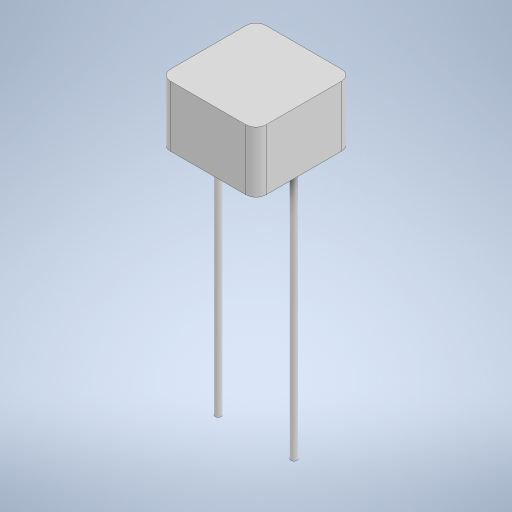
# Autodesk Inventor part: KM6A – H90
Saved by Autodesk Inventor 2024 (Build 280153000, 153)
## iProperties
Created: 2023-12-04
Part Number: KM6A – H90
Material: Типовые
Document SubType Name: Modeling
Designer: SaNe4Ka
Density: 1 g/cm^3
Appearance: По умолчанию
Author: SaNe4Ka
Autodesk Inventor part; units mm, degrees
ref_plane "YZ Plane" through (0, 0, 0) normal (1, 0, 0) x (0, 1, 0)
ref_plane "XZ Plane" through (0, 0, 0) normal (0, 1, 0) x (-1, 0, 0)
ref_plane "XY Plane" through (0, 0, 0) normal (0, 0, 1) x (1, 0, 0)
sketch "Эскиз1" plane through (0, 0, 0) normal (0, 1, 0) x (-1, 0, 0)
  line L0 (5.945, 7.1046) -> (-1.555, 7.1046)
  line L1 (-2.555, 6.1046) -> (-2.555, -1.3954)
  line L2 (-1.555, -2.3954) -> (5.945, -2.3954)
  line L3 (6.945, -1.3954) -> (6.945, 6.1046)
  arc A0 (6.945, 6.1046) -> (5.945, 7.1046) centre (5.945, 6.1046) ccw
  arc A1 (5.945, -2.3954) -> (6.945, -1.3954) centre (5.945, -1.3954) ccw
  arc A2 (-2.555, -1.3954) -> (-1.555, -2.3954) centre (-1.555, -1.3954) ccw
  arc A3 (-1.555, 7.1046) -> (-2.555, 6.1046) centre (-1.555, 6.1046) ccw
  point P0 (0, 0)
  point P1 (-2.555, -2.3954)
  point P2 (-2.555, 7.1046)
  point P3 (6.945, -2.3954)
  dimension "d0" = 9.5
  dimension "d1" = 9.5
  dimension "d2" = 1
  constraints: 8 end point, 8 point on circle, 8 tangent, 6 point on line, 4 centre point, 3 equal radius, 2 parallel, 1 horizontal, 1 perpendicular
  measures "d0" distance of point (6.945, -2.395) point (-2.555, -2.395)
  measures "d1" distance of point (-2.555, -2.395) point (-2.555, 7.105)
  measures "d2" radius of A0
extrude "Выдавливание1" add sketch "Эскиз1" along normal blind 6
sketch "Эскиз2" plane through (0, 0, 0) normal (0, 1, 0) x (-1, 0, 0)
  arc A0 (6.945, 6.1046) -> (5.945, 7.1046) centre (5.945, 6.1046) ccw projected
  arc A1 (-2.555, -1.3954) -> (-1.555, -2.3954) centre (-1.555, -1.3954) ccw projected
  circle A2 centre (5.945, 2.3546) radius 0.3
  circle A3 centre (-1.555, 2.3546) radius 0.3
  line L0 (5.945, 2.3546) -> (-1.555, 2.3546)
  point P0 (0, 0)
  dimension "d7" = 0.6
  dimension "d8" = 0.6
  constraints: 2 centre point, 2 end point, 1 horizontal
  measures "d7" diameter of A2
  measures "d8" diameter of A3
extrude "Выдавливание2" add sketch "Эскиз2" against normal blind 25
